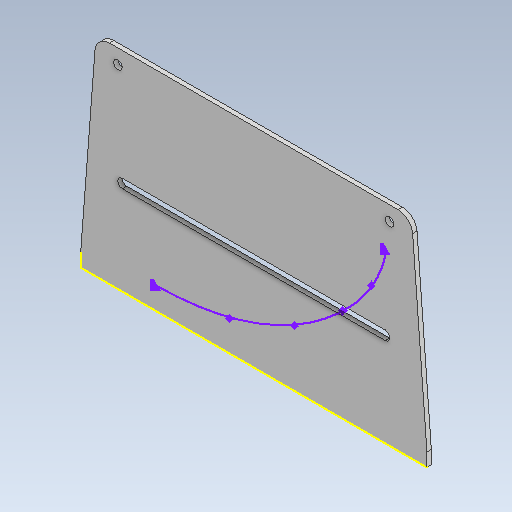
# Autodesk Inventor part: mountback
Saved by Autodesk Inventor 2020 (Build 240168000, 168)
## iProperties
Created: 2021-06-15
Part Number: mountback
Material: Generic
Document SubType Name: Modeling
Designer: Aidan Lee
Density: 1 g/cm^3
Appearance: Default
Author: Aidan Lee
Autodesk Inventor part; units mm, degrees
ref_plane "YZ Plane" through (0, 0, 0) normal (1, 0, 0) x (0, 1, 0)
ref_plane "XZ Plane" through (0, 0, 0) normal (0, 1, 0) x (-1, 0, 0)
ref_plane "XY Plane" through (0, 0, 0) normal (0, 0, 1) x (1, 0, 0)
sketch "Sketch1" plane through (0, 0, 0) normal (0, 0, 1) x (1, 0, 0)
  line L0 (0, 0) -> (237, 0)
  line L1 (10.5075, 133.75) -> (226.4925, 133.75)
  line L2 (10.5075, 133.75) -> (0, 0)
  line L3 (226.4925, 133.75) -> (237, 0)
  circle A0 centre (25.5075, 123.75) radius 3
  line L4 (118.5, 191.0895) -> (118.5, 206.5913) construction
  circle A1 centre (211.4925, 123.75) radius 3
  line L5 (28.5, 54.9) -> (208.5, 54.9) construction
  line L6 (28.5, 51.8) -> (208.5, 51.8)
  line L7 (208.5, 58) -> (28.5, 58)
  arc A2 (28.5, 58) -> (28.5, 51.8) centre (28.5, 54.9) ccw
  arc A3 (208.5, 51.8) -> (208.5, 58) centre (208.5, 54.9) ccw
  point P0 (118.5, 133.75)
  point P1 (118.5, 0)
  point P2 (118.5, 198.8404)
  point P3 (118.5, 54.9)
  dimension "d0" = 237
  dimension "d1" = 215.985
  dimension "d2" = 133.75
  dimension "d3" = 6
  dimension "d4" = 10
  dimension "d5" = 15
  dimension "d8" = 6.2
  dimension "d9" = 81.95
  dimension "d10" = 180
  constraints: 18 end point, 4 centre point, 4 midpoint, 4 point on circle, 4 tangent, 3 horizontal, 3 vertical alignment, 1 parallel, 1 symmetric about line, 1 vertical, 1 other
  measures "d0" distance of L0.start L0.end
  measures "d1" distance of L1.start L1.end
  measures "d2" distance between parallel lines of L0 L1
  measures "d3" diameter of A0
  measures "d4" distance from line of L1 A0.centre
  measures "d5" horizontal distance of A0.centre L1.start
  measures "d8" distance between parallel lines of L6 L7
  measures "d9" distance between parallel lines of L1 L6
  measures "d10" distance of L5.end L5.start
extrude "Extrusion1" add sketch "Sketch1" along normal blind 3
sketch "Sketch2" plane through (0, 0, 3) normal (0, 0, 1) x (1, 0, 0)
  line L0 (0, 0) -> (237, 0)
  line L1 (237, 0) -> (237, -9)
  line L2 (237, -9) -> (0, -9)
  line L3 (0, -9) -> (0, 0)
  dimension "depth" = 9
  constraints: 8 end point, 2 parallel, 1 coincident, 1 horizontal, 1 perpendicular
  measures "depth" distance between parallel lines of L0 L2
extrude "Extrusion2" add sketch "Sketch2" against normal blind 3
fillet "Fillet1" radius 10 2 edges at (226.4925, 133.75, 1.5) (10.5075, 133.75, 1.5)
sketch "Sketch3" plane through (0, 0, 3) normal (0, 0, 1) x (1, 0, 0)
  line L0 (0, 0) -> (0, -9) projected
  line L1 (0, -9) -> (237, -9) projected
  spline S0 degree 4 poles (208.9384, 106.1179) (205.6345, 87.6966) (186.3734, 52.9377) (139.2784, 16.5104) (82.7331, 6.5959) (51.8588, 6.1179) knots 0 0 0 0 0 0.457223 1 1 1 1 1
  point P0 (199.8798, 81.1179)
  point P1 (180.3986, 56.1179)
  point P2 (147.52, 31.1179)
  point P3 (103.0387, 12.8166)
  constraints: 6 other
equation "\"raisedheight\" = 5"
equation "\"geargap\" = 0.2"
body "Solid1"
